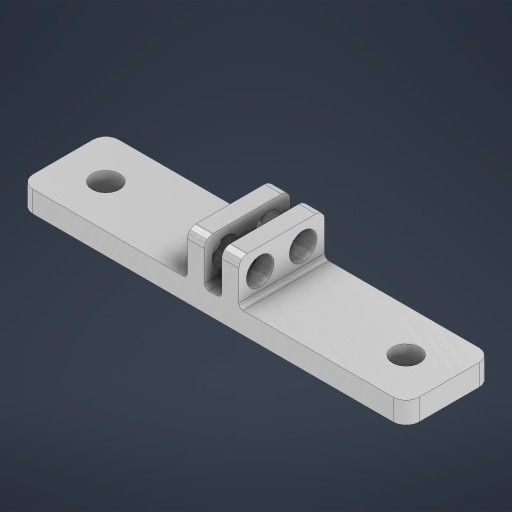
# Autodesk Inventor part: CarbonConnectorPlateConnector
Saved by Autodesk Inventor 2023 (Build 270158000, 158)
## iProperties
Created: 2023-02-23
Part Number: CarbonConnectorPlateConnector
Material: Generic
Document SubType Name: Modeling
Designer: Elias Braun
Density: 1 g/cm^3
Appearance: Machined - Aluminum
Author: Elias Braun
Autodesk Inventor part; units mm, degrees
ref_plane "YZ Plane" through (0, 0, 0) normal (1, 0, 0) x (0, 1, 0)
ref_plane "XZ Plane" through (0, 0, 0) normal (0, 1, 0) x (-1, 0, 0)
ref_plane "XY Plane" through (0, 0, 0) normal (0, 0, 1) x (1, 0, 0)
sketch "Sketch1" plane through (0, 0, 0) normal (0, 1, 0) x (-1, 0, 0)
  line L0 (22.5, 5) -> (-22.5, 5)
  line L1 (-22.5, 5) -> (-22.5, -5)
  line L2 (-22.5, -5) -> (22.5, -5)
  line L3 (22.5, -5) -> (22.5, 5)
  line L4 (22.5, 5) -> (17.5, 5) construction
  line L5 (17.5, 5) -> (17.5, 0) construction
  circle A0 centre (17.5, 0) radius 1.6
  line L6 (0, -5) -> (0, -10.3319) construction
  circle A1 centre (-17.5, 0) radius 1.6
  point P0 (0, 0)
  dimension "d2" = 5
  dimension "d3" = 3.2
  constraints: 14 end point, 2 centre point, 2 parallel, 2 perpendicular, 1 coincident, 1 horizontal, 1 midpoint, 1 point on line, 1 symmetric about line, 1 vertical, 1 other
  measures "d2" distance of L0.start L4.end
  measures "d3" diameter of A0
extrude "Extrusion1" add sketch "Sketch1" along normal blind 2.5
fillet "Fillet1" radius 1.5 4 edges at (-22.5, 1.25, 5) (22.5, 1.25, 5) (22.5, 1.25, -5) (-22.5, 1.25, -5)
sketch "Sketch5" plane through (0, 2.5, 0) normal (0, 1, 0) x (1, 0, 0)
  line L0 (0, 0) -> (-1, 0) construction
  line L1 (0, 0) -> (1, 0) construction
  line L2 (-1, 5) -> (-3, 5)
  line L3 (-3, 5) -> (-3, -5)
  line L4 (-21, -5) -> (21, -5) projected
  line L5 (-3, -5) -> (-1, -5)
  line L6 (-1, -5) -> (-1, 5)
  line L7 (21, 5) -> (-21, 5) projected
  line L8 (0, 0) -> (0, 0.5432) construction
  line L9 (1, 5) -> (3, 5)
  line L10 (3, 5) -> (3, -5)
  line L11 (21, -5) -> (-21, -5)
  line L12 (3, -5) -> (1, -5)
  line L13 (1, -5) -> (1, 5)
  dimension "d33" = 2
  constraints: 24 end point, 6 symmetric about line, 4 point on line, 2 horizontal, 2 vertical, 1 perpendicular
  measures "d33" distance of L2.start L2.end
extrude "Extrusion5" add sketch "Sketch5" along normal blind 5 contours L6 L4 L3 L2 | L7 L10 L4 L13
sketch "Sketch6" plane through (3, 2.5, 5) normal (1, 0, 0) x (0, 0, -1)
  line L0 (10, -2.5) -> (10, 0) construction
  line L1 (-0.0046, 4.9481) -> (10, 0) construction
  line L2 (10, 5) -> (0, 5) construction
  line L3 (10, 5) -> (0, 0) construction
  line L4 (4.9728, 2.4864) -> (4.9728, 3.4864) construction
  line L5 (4.9728, 2.4864) -> (2.4728, 2.4864) construction
  circle A0 centre (2.4728, 2.4864) radius 1.6
  circle A1 centre (7.4728, 2.4864) radius 1.6
  point P0 (5, -2.5)
  dimension "d38" = 3.2
  constraints: 8 end point, 2 centre point, 2 point on line, 1 coincident, 1 horizontal, 1 symmetric about line, 1 vertical, 1 other
  measures "d38" diameter of A0
extrude "Extrusion6" cut sketch "Sketch6" against normal blind 6
fillet "Fillet6" radius 1 4 edges at (-2, 7.5, 5) (2, 7.5, 5) (2, 7.5, -5) (-2, 7.5, -5)
fillet "Fillet7" radius 0.5 4 edges at (-3, 2.5, 0) (-1, 2.5, 0) (3, 2.5, 0) (1, 2.5, 0)
body "Solid1"
